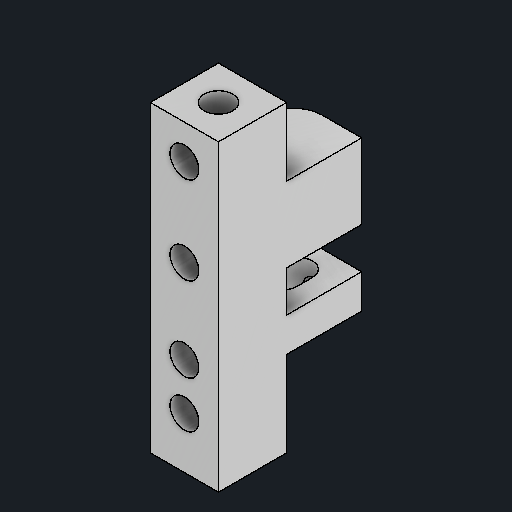
# Autodesk Inventor part: A Idler
Saved by Autodesk Inventor 2026.2 (Build 302298000, 298)
## iProperties
Created: 2025-04-15
Part Number: A Idler
Material: Aluminum 6061
Document SubType Name: Modeling
Designer: Joshua Eah
Density: 2.7 g/cm^3
Appearance: Machined - Aluminum
Author: Joshua Eah
Autodesk Inventor part; units mm, degrees
ref_plane "YZ Plane" through (0, 0, 0) normal (1, 0, 0) x (0, 1, 0)
ref_plane "XZ Plane" through (0, 0, 0) normal (0, 1, 0) x (-1, 0, 0)
ref_plane "XY Plane" through (0, 0, 0) normal (0, 0, 1) x (1, 0, 0)
sketch "Base Profile" plane through (0, 0, 0) normal (0, 1, 0) x (-1, 0, 0)
  line L0 (0, 0) -> (15, 0)
  line L1 (15, 0) -> (15, -15)
  line L2 (15, -15) -> (0, -15)
  line L3 (0, -15) -> (0, 0)
  line L4 (15, 0) -> (31.5, 0)
  line L5 (31.5, 0) -> (31.5, -15)
  line L6 (31.5, -15) -> (15, -15)
  line L7 (15, -15) -> (15, 0)
  dimension "d164" = 15
  dimension "d165" = 15
  dimension "d166" = 16.5
  dimension "d167" = 15
  constraints: 16 end point, 4 parallel, 2 horizontal, 2 perpendicular, 2 point on line
  measures "d164" distance of L1.end L2.end
  measures "d165" distance of L0.end L1.end
  measures "d166" distance of L5.end L6.end
  measures "d167" distance of L4.end L5.end
extrude "Stock" add sketch "Base Profile" against normal blind 33
extrude "Top Extrusion Post" add sketch "Base Profile" along normal blind 15 contours L0 L1 L2 L3
extrude "Lower Extrusion Post" add sketch "Base Profile" against normal blind 18.75 from surface at -33 contours L0 L1 L2 L3
sketch "Sketch27" plane through (0, -33, -15) normal (0, 0, -1) x (-1, 0, 0)
  line L0 (0, -18.75) -> (0, 48) projected
  line L1 (31.5, 0) -> (15, 0) projected
  line L2 (31.5, 33) -> (31.5, 0) projected
  line L3 (15, 33) -> (31.5, 33) projected
  line L4 (15, 33) -> (15, 48) projected
  line L5 (0, 48) -> (15, 48) projected
  line L6 (0, 16.5) -> (31.5, 16.5)
  line L7 (0, 7.5) -> (31.5, 7.5)
  line L8 (15, 33) -> (15, 0)
  line L9 (0, -18.75) -> (15, -18.75) projected
  line L10 (15, 0) -> (15, -18.75) projected
  point P0 (15, 16.5)
  point P1 (15, 7.5)
  dimension "d247" = 16.5
  dimension "d290" = 7.5
  constraints: 6 end point, 4 point on line, 2 perpendicular, 1 horizontal, 1 midpoint
  measures "d247" distance between parallel lines of L1 L6
  measures "d290" distance between parallel lines of L1 L7
extrude "Lower Half Cut" cut sketch "Sketch27" against normal through all contours L8 L6 L2 L7
sketch "Bottom Profile" plane through (-35, -33, -15) normal (0, -1, 0) x (1, 0, 0)
  line L0 (13.5, 7.5) -> (10, 7.5) construction
  line L1 (13.5, 10.675) -> (10, 10.675)
  line L2 (10, 4.325) -> (13.5, 4.325)
  arc A0 (13.5, 4.325) -> (13.5, 10.675) centre (13.5, 7.5) ccw
  arc A1 (10, 10.675) -> (10, 4.325) centre (10, 7.5) ccw
  line L3 (3.5, 15) -> (3.5, 0) projected
  line L4 (35, 15) -> (3.5, 15) projected
  point P0 (11.75, 7.5)
  dimension "d291" = 3.5
  dimension "d292" = 6.35
  dimension "d293" = 6.5
  dimension "d294" = 7.5
  constraints: 8 end point, 4 point on circle, 4 tangent, 2 centre point, 1 horizontal, 1 midpoint, 1 parallel
  measures "d291" distance of L0.start L0.end
  measures "d292" diameter of A1
  measures "d293" distance from line of L3 L0.end
  measures "d294" distance from line of L4 L0.end
extrude "Slot Cut" cut sketch "Bottom Profile" against normal blind 24
sketch "Front Hole Pattern" plane through (0, -33, 0) normal (1, 0, 0) x (0, 0, -1)
  line L0 (0, 0) -> (0, 48) projected
  circle A0 centre (7.5, 40.5) radius 3.175
  line L1 (0, 48) -> (15, 48) projected
  circle A1 centre (7.5, 21.25) radius 3.175
  line L2 (15, 0) -> (0, 0) projected
  circle A2 centre (7.5, -7.5) radius 3.175
  circle A3 centre (7.5, 2.75) radius 3.175
  dimension "d317" = 6.35
  dimension "d318" = 7.5
  dimension "d319" = 7.5
  dimension "d354" = 6.35
  dimension "d356" = 21.25
  dimension "d369" = 6.35
  dimension "d370" = 7.5
  dimension "d371" = 6.35
  dimension "d372" = 2.75
  constraints: 4 centre point, 3 vertical alignment
  measures "d317" diameter of A0
  measures "d318" distance from line of A0.centre L0
  measures "d319" distance from line of A0.centre L1
  measures "d354" diameter of A1
  measures "d356" distance from line of L2 A1.centre
  measures "d369" diameter of A2
  measures "d370" distance from line of A2.centre L2
  measures "d371" diameter of A3
  measures "d372" distance from line of L2 A3.centre
hole "Front Adjustment Hole" at (0, -11.75, -7.5) at (0, -30.25, -7.5) direction (-1, 0, 0) diameter 3.2004 end through all start extended yes counterbore diameter 6.35 counterbore depth 10.675 clearance for "Socket Head Cap Screw" size "M3" standard "Ansi Metric M Profile"
hole "Front Mounting Hole" at (0, 7.5, -7.5) at (0, -40.5, -7.5) direction (-1, 0, 0) diameter 3.2004 end through all start extended yes counterbore diameter 6.35 counterbore depth 10.675 clearance for "Socket Head Cap Screw" size "M3" standard "Ansi Metric M Profile"
sketch "Sketch33" plane through (0, 15, 0) normal (0, 1, 0) x (1, 0, 0)
  line L0 (-15, 15) -> (-15, 0) projected
  line L1 (-15, 0) -> (0, 0) projected
  line L2 (0, 0) -> (0, 15) projected
  line L3 (0, 15) -> (-15, 15) projected
  circle A0 centre (-7.5, 7.5) radius 3.175
  dimension "d340" = 6.35
  dimension "d341" = 7.5
  dimension "d342" = 7.5
  constraints: 1 centre point
  measures "d340" diameter of A0
  measures "d341" distance from line of A0.centre L2
  measures "d342" distance from line of A0.centre L1
hole "Top Mounting Hole" at (-7.5, 15, -7.5) direction (0, -1, 0) diameter 3.2004 end through all start extended yes counterbore diameter 6.35 counterbore depth 61.674 clearance for "Socket Head Cap Screw" size "M3" standard "Ansi Metric M Profile"
fillet "Fillet2" radius 6.35 2 edges at (-31.5, -29.25, 0) (-31.5, -8.25, 0)
equation "\"d164\" = extrusionWidth"
equation "\"d165\" = extrusionWidth"
equation "\"d166\" = idlerLength"
equation "\"d167\" = d165"
equation "\"d168\" = extrusionOffset"
equation "\"extrusionWidth\" = 15"
equation "\"idlerLength\" = 16.5"
equation "\"bearingOffsetFromBottom\" = 7.5"
equation "\"extrusionOffset\" = 33"
equation "\"bearingStackHeight\" = 9"
equation "\"bearingSlotLength\" = 3.5"
equation "\"bearingClearance\" = 13"
equation "\"pinSupportLength\" = 2"
body "Solid2"
